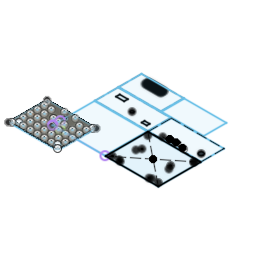
script OS 25 v11 (Autodesk Fusion 360 design; units mm, degrees)
Autodesk Fusion 360 part; units mm, degrees
(part 1 of 6)
sketch "top content" plane through (0, 0, 0) normal (0, 0, 1) x (1, 0, 0)
  circle A0 centre (59.5, 109.5) radius 1.5
  circle A1 centre (59.5, 78.5) radius 1.5
  circle A2 centre (90.5, 109.5) radius 1.5
  line L0 (0, 120) -> (150, 120) construction
  line L1 (150, 120) -> (150, 0) construction
  line L2 (150, 0) -> (0, 0) construction
  circle A3 centre (20, 20) radius 6.4
  circle A4 centre (75, 60) radius 1.588
  circle A5 centre (90.5, 78.5) radius 1.5
  circle A6 centre (75, 94) radius 11
  line L3 (0, 0) -> (0, 120) construction
  line L4 (1.75, 0) -> (22.5, 0)
  line L5 (0, 1.75) -> (0, 22.5)
  line L6 (0, 60) -> (150, 60) construction
  line L7 (75, 120) -> (75, 0) construction
  circle A7 centre (130, 20) radius 6.4
  point P0 (75, 60)
  point P1 (75, 60)
  dimension "d2090" = 31
  dimension "d2091" = 31
  dimension "d2092" = 150
  dimension "d2093" = 120
  dimension "d2094" = 12.8
  dimension "d2096" = 3
  dimension "d2104" = 15.5
  dimension "d2105" = 15.5
  dimension "d5914" = 22
  dimension "d5917" = 40
  dimension "d5918" = 55
  dimension "d5919" = 34
  constraint perpendicular L0 L1
  constraint parallel L0 L2
  constraint parallel L1 L3
  constraint coincident P1 P0
  constraint horizontal L2
  constraint collinear L2 L4
  constraint collinear L3 L5
  constraint midpoint L3 L6.start
  constraint midpoint L1 L6.end
  constraint midpoint L0 L7.start
  constraint midpoint L2 L7.end
  constraint coincident A6.centre L7
  constraint symmetric A3 L7 A7
  measures "d2092" distance of L0.start L0.end
  measures "d2093" distance of L0.start L2.end
  measures "d2094" diameter of A3
  measures "d2096" diameter of A1
  measures "d2104" horizontal distance of A6.centre A2.centre
  measures "d2105" vertical distance of A6.centre A5.centre
  measures "d5914" diameter of A6
  measures "d5917" distance of A3.centre L6
  measures "d5918" distance of A3.centre L7
  measures "d5919" distance of A6.centre L6
sketch "platform content" plane through (0, 0, 0) normal (0, 0, 1) x (1, 0, 0) in component "platform"
  circle A0 centre (55, -40) radius 6.4
  line L0 (-70, -50) -> (-70, 50)
  line L1 (-65, 55) -> (65, 55)
  line L2 (-70, 0) -> (70, 0) construction
  circle A1 centre (-15.5, 49.5) radius 1.5
  line L3 (70, 50) -> (70, -50)
  line L4 (65, -55) -> (-65, -55)
  line L5 (0, 55) -> (0, -55) construction
  circle A2 centre (-55, -40) radius 6.4
  circle A3 centre (15.5, 18.5) radius 1.5
  circle A4 centre (-15.5, 18.5) radius 1.5
  circle A5 centre (0, 34) radius 6.4
  circle A6 centre (15.5, 49.5) radius 1.5
  arc A7 (-70, -50) -> (-65, -55) centre (-65, -50) ccw
  arc A8 (65, -55) -> (70, -50) centre (65, -50) ccw
  arc A9 (70, 50) -> (65, 55) centre (65, 50) ccw
  arc A10 (-65, 55) -> (-70, 50) centre (-65, 50) ccw
  circle A11 centre (0, 0) radius 1.005
  circle A12 centre (0, -3) radius 1.5
  circle A13 centre (-40, -43) radius 1.5
  circle A14 centre (-60, -23) radius 1.5
  circle A15 centre (-60, -3) radius 1.5
  circle A16 centre (40, -43) radius 1.5
  circle A17 centre (0, -23) radius 1.5
  circle A18 centre (-20, -3) radius 1.5
  circle A19 centre (40, -3) radius 1.5
  circle A20 centre (60, -3) radius 1.5
  circle A21 centre (60, -23) radius 1.5
  circle A22 centre (-20, -43) radius 1.5
  circle A23 centre (20, -43) radius 1.5
  circle A24 centre (-40, -3) radius 1.5
  circle A25 centre (20, -3) radius 1.5
  circle A26 centre (-60, 17) radius 1.5
  circle A27 centre (-40, 17) radius 1.5
  circle A28 centre (0, 17) radius 1.5
  circle A29 centre (40, 17) radius 1.5
  circle A30 centre (60, 17) radius 1.5
  circle A31 centre (-60, 37) radius 1.5
  circle A32 centre (-40, 37) radius 1.5
  circle A33 centre (40, 37) radius 1.5
  circle A34 centre (60, 37) radius 1.5
  circle A35 centre (0, -43) radius 1.5
  circle A36 centre (-40, -23) radius 1.5
  circle A37 centre (-20, -23) radius 1.5
  circle A38 centre (20, -23) radius 1.5
  circle A39 centre (40, -23) radius 1.5
  circle A40 centre (-65, 50) radius 1.5
  circle A41 centre (65, 50) radius 1.5
  circle A42 centre (65, -50) radius 1.5
  circle A43 centre (-65, -50) radius 1.5
  point P0 (-70, -55)
  point P1 (70, 55)
  point P2 (-70, 55)
  dimension "d5927" = 31
  dimension "d5928" = 31
  dimension "d5929" = 140
  dimension "d5930" = 110
  dimension "d5931" = 12.8
  dimension "d5932" = 3
  dimension "d5933" = 15.5
  dimension "d5934" = 15.5
  dimension "d5935" = 12.8
  dimension "d5936" = 40
  dimension "d5937" = 55
  dimension "d5938" = 34
  dimension "d5939" = 5
  dimension "d5940" = 5
  dimension "d5941" = 5
  dimension "d5942" = 5
  dimension "d5943" = 2.01
  dimension "d5948" = 70
  dimension "d5959" = 3
  dimension "d5960" = 3
  dimension "d5961" = 37
  dimension "d5962" = 37
  dimension "d5965" = 20
  dimension "d5966" = 20
  dimension "d5967" = 3
  dimension "d5968" = 3
  dimension "d5969" = 3
  dimension "d5970" = 3
  constraint perpendicular L1 L3
  constraint parallel L1 L4
  constraint parallel L0 L3
  constraint horizontal L4
  constraint coincident A5.centre L5
  constraint symmetric A0 L5 A2
  constraint midpoint L5 A11.centre
  constraint coincident L2.start L0
  constraint coincident L5.end L4
  constraint coincident P0 L0
  constraint coincident P0 L4
  constraint tangent L0 A7
  constraint tangent L4 A7
  constraint coincident L2.end L3
  constraint tangent L4 A8
  constraint tangent L3 A8
  constraint coincident L5.start L1
  constraint coincident P1 L1
  constraint coincident P1 L3
  constraint tangent L1 A9
  constraint tangent L3 A9
  constraint coincident P2 L1
  constraint coincident P2 L0
  constraint tangent L1 A10
  constraint tangent L0 A10
  constraint coincident A11.centre origin
  constraint vertical L5
  constraint horizontal L2
  constraint coincident L2 A11.centre
  constraint coincident L5 A12.centre
  constraint concentric A10 A40
  constraint concentric A9 A41
  constraint concentric A8 A42
  constraint concentric A7 A43
  measures "d5929" distance of P1 P2
  measures "d5930" distance of P0 P2
  measures "d5931" diameter of A2
  measures "d5932" diameter of A4
  measures "d5933" horizontal distance of A6.centre A5.centre
  measures "d5934" vertical distance of A3.centre A5.centre
  measures "d5935" diameter of A5
  measures "d5936" distance of A2.centre L2
  measures "d5937" distance of A2.centre L5
  measures "d5938" distance of A5.centre L2
  measures "d5939" radius of A7
  measures "d5940" radius of A8
  measures "d5941" radius of A9
  measures "d5942" radius of A10
  measures "d5943" diameter of A11
  measures "d5948" distance of L3 L5
  measures "d5959" diameter of A12
  measures "d5960" distance of L2 A12.centre
  measures "d5961" vertical distance of A0.centre A12.centre
  measures "d5962" distance of A5.centre A12.centre
  measures "d5967" diameter of A40
  measures "d5968" diameter of A41
  measures "d5969" diameter of A42
  measures "d5970" diameter of A43
sketch "bottom content" plane through (0, 0, 0) normal (0, 0, 1) x (1, 0, 0)
  line L0 (302.01, 120) -> (152.01, 120)
  line L1 (152.01, 120) -> (152.01, 0)
  line L2 (152.01, 0) -> (302.01, 0)
  line L3 (302.01, 0) -> (302.01, 120)
  line L4 (302.01, 120) -> (152.01, 0) construction
  line L5 (152.01, 120) -> (302.01, 0) construction
  circle A0 centre (180.01, 10) radius 1
  circle A1 centre (161.535, 9.525) radius 1.005
  line L6 (150, 0) -> (0, 0)
  circle A2 centre (186.01, 7.175) radius 1
  circle A3 centre (268.01, 7.175) radius 1
  circle A4 centre (186.01, 69.175) radius 1
  circle A5 centre (268.01, 69.175) radius 1
  point P0 (227.01, 60)
  point P1 (274.01, 10)
  point P2 (180.01, 58)
  point P3 (274.01, 58)
  point P4 (292.485, 110.475)
  point P5 (292.485, 9.525)
  point P6 (161.535, 110.475)
  point P7 (292.485, 110.475)
  dimension "d3674" = 150
  dimension "d3675" = 120
  dimension "d3676" = 2
  dimension "d3677" = 10
  dimension "d3678" = 47
  dimension "d3681" = 94
  dimension "d3682" = 48
  dimension "d3683" = 2.01
  dimension "d3684" = 9.525
  dimension "d3685" = 9.525
  dimension "d3687" = 360
  dimension "d3690" = 130.95
  dimension "d3691" = 100.95
  dimension "d3731" = 152.01
  dimension "d5973" = 2
  dimension "d5974" = 7.175
  dimension "d5977" = 82
  dimension "d5978" = 62
  dimension "d5979" = 41
  constraint horizontal L0
  constraint perpendicular L0 L1
  constraint parallel L0 L2
  constraint parallel L1 L3
  constraint coincident L4 P0
  constraint coincident L5 P0
  constraint collinear L2 L6
  measures "d3674" distance of L1.end L2.end
  measures "d3675" distance of L0.start L2.end
  measures "d3676" diameter of A0
  measures "d3677" distance of L2 A0.centre
  measures "d3678" horizontal distance of P0 A0.centre
  measures "d3683" diameter of A1
  measures "d3684" distance of L2 A1.centre
  measures "d3685" distance of L1 A1.centre
  measures "d3731" distance of L6.end L1
  measures "d5973" diameter of A2
  measures "d5974" distance of L2 A2.centre
  measures "d5979" horizontal distance of P0 A2.centre
sketch "back content" plane through (0, 0, 0) normal (0, 0, 1) x (1, 0, 0)
  line L0 (152.01, 187.01) -> (302.01, 187.01) construction
  line L1 (302.01, 187.01) -> (302.01, 122.01) construction
  line L2 (302.01, 122.01) -> (152.01, 122.01) construction
  line L3 (152.01, 122.01) -> (152.01, 187.01) construction
  circle A0 centre (282.01, 142.01) radius 5.6
  line L4 (0, 0) -> (0, 120)
  line L5 (206.01, 128.51) -> (196.01, 128.51)
  line L6 (196.01, 128.51) -> (196.01, 138.51)
  line L7 (196.01, 138.51) -> (206.01, 138.51)
  line L8 (206.01, 138.51) -> (206.01, 128.51)
  line L9 (206.01, 128.51) -> (196.01, 138.51) construction
  line L10 (196.01, 128.51) -> (206.01, 138.51) construction
  line L11 (186.01, 128.51) -> (246, 128.51) construction
  line L12 (224.51, 139.51) -> (212.51, 139.51)
  line L13 (212.51, 139.51) -> (212.51, 128.51)
  line L14 (212.51, 128.51) -> (224.51, 128.51)
  line L15 (224.51, 128.51) -> (224.51, 139.51)
  line L16 (224.51, 139.51) -> (212.51, 128.51) construction
  line L17 (212.51, 139.51) -> (224.51, 128.51) construction
  line L18 (248.71, 128.51) -> (233.71, 128.51)
  line L19 (233.71, 128.51) -> (233.71, 131.01)
  line L20 (233.71, 131.01) -> (248.71, 131.01)
  line L21 (248.71, 131.01) -> (248.71, 128.51)
  line L22 (248.71, 128.51) -> (233.71, 131.01) construction
  line L23 (233.71, 128.51) -> (248.71, 131.01) construction
  point P0 (22.5, 0)
  point P1 (201.01, 133.51)
  point P2 (218.51, 134.01)
  point P3 (241.21, 129.76)
  dimension "d381" = 150
  dimension "d382" = 65
  dimension "d387" = 11.2
  dimension "d388" = 20
  dimension "d389" = 20
  dimension "d3694" = 152.01
  dimension "d3695" = 122.01
  dimension "d5984" = 6.5
  dimension "d5985" = 10
  dimension "d5986" = 10
  dimension "d5987" = 15
  dimension "d5988" = 12
  dimension "d5989" = 32.5
  dimension "d5990" = 11
  dimension "d5991" = 15
  dimension "d5992" = 2.5
  dimension "d5993" = 55.2
  dimension "d5995" = 34
  constraint horizontal L0
  constraint horizontal L2
  constraint vertical L3
  constraint vertical L1
  constraint horizontal L5
  constraint perpendicular L5 L6
  constraint parallel L5 L7
  constraint parallel L6 L8
  constraint coincident L9 P1
  constraint coincident L10 P1
  constraint perpendicular L6 L11
  constraint collinear L5 L11
  constraint horizontal L12
  constraint perpendicular L12 L13
  constraint parallel L12 L14
  constraint parallel L13 L15
  constraint coincident L16 P2
  constraint coincident L17 P2
  constraint collinear L11 L14
  constraint horizontal L18
  constraint perpendicular L18 L19
  constraint parallel L18 L20
  constraint parallel L19 L21
  constraint coincident L22 P3
  constraint coincident L23 P3
  constraint collinear L11 L18
  measures "d381" distance of L0.start L0.end
  measures "d382" distance of L0.start L2.end
  measures "d387" diameter of A0
  measures "d388" distance of L2 A0.centre
  measures "d389" distance of L1 A0.centre
  measures "d3694" distance of L3 L4
  measures "d3695" distance of L2 P0
  measures "d5984" distance of L2 L11
  measures "d5985" distance of L5.end L6.end
  measures "d5986" distance of L6.end L7.end
  measures "d5987" horizontal distance of P1 L11.start
  measures "d5988" distance of L13.end L14.end
  measures "d5989" horizontal distance of L11.start P2
  measures "d5990" distance of L12.start L14.end
  measures "d5991" distance of L19.end L20.end
  measures "d5992" distance of L18.start L20.end
  measures "d5993" horizontal distance of L11.start P3
  measures "d5995" horizontal distance of L2.end L11.start
sketch "front content" plane through (0, 0, 0) normal (0, 0, 1) x (1, 0, 0)
  line L0 (20, 172.01) -> (43, 172.01)
  line L1 (43, 172.01) -> (43, 161.51)
  line L2 (43, 161.51) -> (20, 161.51)
  line L3 (20, 161.51) -> (20, 172.01)
  circle A0 centre (80, 147.01) radius 3.5
  line L4 (120.5, 142.21) -> (135, 142.21)
  line L5 (135, 142.21) -> (135, 134.01)
  line L6 (135, 134.01) -> (120.5, 134.01)
  line L7 (120.5, 134.01) -> (120.5, 142.21)
  line L8 (0, 187.01) -> (150, 187.01) construction
  line L9 (150, 187.01) -> (150, 122.01) construction
  line L10 (150, 122.01) -> (0, 122.01) construction
  line L11 (0, 122.01) -> (0, 187.01) construction
  line L12 (150, 0) -> (0, 0)
  line L13 (0, 1.75) -> (0, 22.5)
  dimension "d332" = 23
  dimension "d333" = 10.5
  dimension "d336" = 7
  dimension "d339" = 14.5
  dimension "d340" = 8.2
  dimension "d371" = 150
  dimension "d372" = 65
  dimension "d374" = 20
  dimension "d376" = 15
  dimension "d377" = 12
  dimension "d378" = 15
  dimension "d379" = 25
  dimension "d380" = 70
  dimension "d3693" = 122.01
  constraint horizontal L0
  constraint vertical L1
  constraint horizontal L2
  constraint vertical L3
  constraint horizontal L4
  constraint vertical L5
  constraint horizontal L6
  constraint vertical L7
  constraint horizontal L8
  constraint vertical L9
  constraint horizontal L10
  constraint vertical L11
  constraint collinear L11 L13
  measures "d332" distance of L0.start L0.end
  measures "d333" distance of L0.start L2.end
  measures "d336" diameter of A0
  measures "d339" distance of L4.start L4.end
  measures "d340" distance of L4.start L6.end
  measures "d371" distance of L8.start L8.end
  measures "d372" distance of L8.start L10.end
  measures "d374" distance of L3 L11
  measures "d376" distance of L0 L8
  measures "d377" distance of L6 L10
  measures "d378" distance of L5 L9
  measures "d379" distance of A0.centre L10
  measures "d380" distance of A0.centre L9
  measures "d3693" distance of L10.end L12
sketch "left content" plane through (0, 0, 0) normal (0, 0, 1) x (1, 0, 0)
  line L0 (120, 254.02) -> (120, 189.02) construction
  line L1 (120, 189.02) -> (0, 189.02) construction
  line L2 (0, 189.02) -> (0, 254.02) construction
  line L3 (0, 254.02) -> (120, 254.02) construction
  line L4 (0, 1.75) -> (0, 22.5)
  circle A0 centre (30, 234.02) radius 1.005
  circle A1 centre (30, 239.02) radius 1.005
  circle A2 centre (30, 244.02) radius 1.005
  circle A3 centre (35, 234.02) radius 1.005
  circle A4 centre (40, 234.02) radius 1.005
  circle A5 centre (45, 234.02) radius 1.005
  circle A6 centre (50, 234.02) radius 1.005
  circle A7 centre (55, 234.02) radius 1.005
  circle A8 centre (60, 234.02) radius 1.005
  circle A9 centre (65, 234.02) radius 1.005
  circle A10 centre (70, 234.02) radius 1.005
  circle A11 centre (75, 234.02) radius 1.005
  circle A12 centre (35, 239.02) radius 1.005
  circle A13 centre (40, 239.02) radius 1.005
  circle A14 centre (45, 239.02) radius 1.005
  circle A15 centre (50, 239.02) radius 1.005
  circle A16 centre (55, 239.02) radius 1.005
  circle A17 centre (60, 239.02) radius 1.005
  circle A18 centre (65, 239.02) radius 1.005
  circle A19 centre (70, 239.02) radius 1.005
  circle A20 centre (75, 239.02) radius 1.005
  circle A21 centre (35, 244.02) radius 1.005
  circle A22 centre (40, 244.02) radius 1.005
  circle A23 centre (45, 244.02) radius 1.005
  circle A24 centre (50, 244.02) radius 1.005
  circle A25 centre (55, 244.02) radius 1.005
  circle A26 centre (60, 244.02) radius 1.005
  circle A27 centre (65, 244.02) radius 1.005
  circle A28 centre (70, 244.02) radius 1.005
  circle A29 centre (75, 244.02) radius 1.005
  point P0 (22.5, 0)
  dimension "d2844" = 65
  dimension "d2845" = 120
  dimension "d3696" = 189.02
  dimension "d3712" = 2.01
  dimension "d3715" = 5
  dimension "d3716" = 5
  dimension "d3717" = 30
  dimension "d3718" = 10
  constraint coincident L0.end L1.start
  constraint coincident L2.end L3.start
  constraint collinear L2 L4
  constraint horizontal L3
  constraint horizontal L1
  measures "d2844" distance of L2.end L1.end
  measures "d2845" distance of L0 L2
  measures "d3696" distance of L1 P0
  measures "d3712" diameter of A0
  measures "d3717" distance of L2 A0.centre
  measures "d3718" distance of L3 A2.centre
sketch "right content" plane through (0, 0, 0) normal (0, 0, 1) x (1, 0, 0)
  circle A0 centre (157.01, 239.02) radius 1.005
  line L0 (122.01, 189.02) -> (122.01, 254.02) construction
  circle A1 centre (162.01, 244.02) radius 1.005
  circle A2 centre (172.01, 244.02) radius 1.005
  circle A3 centre (162.01, 234.02) radius 1.005
  circle A4 centre (192.01, 239.02) radius 1.005
  circle A5 centre (157.01, 234.02) radius 1.005
  circle A6 centre (152.01, 244.02) radius 1.005
  line L1 (122.01, 254.02) -> (242.01, 254.02) construction
  circle A7 centre (197.01, 239.02) radius 1.005
  circle A8 centre (167.01, 234.02) radius 1.005
  circle A9 centre (187.01, 244.02) radius 1.005
  circle A10 centre (152.01, 234.02) radius 1.005
  circle A11 centre (162.01, 239.02) radius 1.005
  line L2 (242.01, 254.02) -> (242.01, 189.02) construction
  circle A12 centre (197.01, 244.02) radius 1.005
  line L3 (242.01, 189.02) -> (122.01, 189.02) construction
  circle A13 centre (197.01, 234.02) radius 1.005
  circle A14 centre (182.01, 239.02) radius 1.005
  circle A15 centre (187.01, 239.02) radius 1.005
  circle A16 centre (172.01, 239.02) radius 1.005
  circle A17 centre (182.01, 244.02) radius 1.005
  circle A18 centre (177.01, 239.02) radius 1.005
  circle A19 centre (152.01, 239.02) radius 1.005
  circle A20 centre (177.01, 244.02) radius 1.005
  circle A21 centre (167.01, 244.02) radius 1.005
  circle A22 centre (157.01, 244.02) radius 1.005
  circle A23 centre (192.01, 244.02) radius 1.005
  circle A24 centre (187.01, 234.02) radius 1.005
  circle A25 centre (192.01, 234.02) radius 1.005
  circle A26 centre (177.01, 234.02) radius 1.005
  circle A27 centre (182.01, 234.02) radius 1.005
  circle A28 centre (167.01, 239.02) radius 1.005
  circle A29 centre (172.01, 234.02) radius 1.005
  dimension "d3723" = 5
  dimension "d3724" = 5
  dimension "d3726" = 120
  dimension "d3727" = 2.01
  dimension "d3728" = 30
  dimension "d3729" = 10
  dimension "d3730" = 65
  dimension "d5980" = 189.02
  dimension "d5981" = 122.01
  constraint coincident L2.end L3.start
  constraint coincident L0.end L1.start
  constraint horizontal L1
  constraint horizontal L3
  constraint vertical L2
  measures "d3726" distance of L0 L2
  measures "d3727" diameter of A10
  measures "d3728" distance of A10.centre L0
  measures "d3729" distance of A6.centre L1
  measures "d3730" distance of L1 L3
  measures "d5980" vertical distance of origin L0.start
  measures "d5981" horizontal distance of origin L0.end
sketch "b  stock" plane through (0, 0, 0) normal (0, 0, 1) x (1, 0, 0)
  line L0 (0, 0) -> (304.8, 0)
  line L1 (304.8, 0) -> (304.8, 609.6)
  line L2 (304.8, 609.6) -> (0, 609.6)
  line L3 (0, 609.6) -> (0, 0)
extrude "b  stock body extrude" add sketch "b  stock" along normal blind 3.175 makes body 1
sketch "b  layout" plane through (0, 0, 0) normal (0, 0, 1) x (1, 0, 0)
  line L0 (0, 0) -> (150, 0)
  line L1 (150, 0) -> (150, 120)
  line L2 (150, 120) -> (0, 120)
  line L3 (0, 120) -> (0, 0)
  line L4 (152.01, 0) -> (302.01, 0)
  line L5 (302.01, 0) -> (302.01, 120)
  line L6 (302.01, 120) -> (152.01, 120)
  line L7 (152.01, 120) -> (152.01, 0)
  line L8 (0, 122.01) -> (150, 122.01)
  line L9 (150, 122.01) -> (150, 187.01)
  line L10 (150, 187.01) -> (0, 187.01)
  line L11 (0, 187.01) -> (0, 122.01)
  line L12 (152.01, 122.01) -> (302.01, 122.01)
  line L13 (302.01, 122.01) -> (302.01, 187.01)
  line L14 (302.01, 187.01) -> (152.01, 187.01)
  line L15 (152.01, 187.01) -> (152.01, 122.01)
  line L16 (0, 189.02) -> (120, 189.02)
  line L17 (120, 189.02) -> (120, 254.02)
  line L18 (120, 254.02) -> (0, 254.02)
  line L19 (0, 254.02) -> (0, 189.02)
  line L20 (122.01, 189.02) -> (242.01, 189.02)
  line L21 (242.01, 189.02) -> (242.01, 254.02)
  line L22 (242.01, 254.02) -> (122.01, 254.02)
  line L23 (122.01, 254.02) -> (122.01, 189.02)
sketch "b top lines" plane through (0, 0, 0) normal (0, 0, 1) x (1, 0, 0) in component "b top component"
  line L0 (0, 0) -> (10.08, 0)
  line L1 (10.08, 0) -> (10.08, 3.175)
  line L2 (10.08, 3.175) -> (19.92, 3.175)
  line L3 (19.92, 3.175) -> (19.92, 0)
  line L4 (19.92, 0) -> (30.08, 0)
  line L5 (30.08, 0) -> (30.08, 3.175)
  line L6 (30.08, 3.175) -> (39.92, 3.175)
  line L7 (39.92, 3.175) -> (39.92, 0)
  line L8 (39.92, 0) -> (50.08, 0)
  line L9 (50.08, 0) -> (50.08, 3.175)
  line L10 (50.08, 3.175) -> (59.92, 3.175)
  line L11 (59.92, 3.175) -> (59.92, 0)
  line L12 (59.92, 0) -> (70.08, 0)
  line L13 (70.08, 0) -> (70.08, 3.175)
  line L14 (70.08, 3.175) -> (79.92, 3.175)
  line L15 (79.92, 3.175) -> (79.92, 0)
  line L16 (79.92, 0) -> (90.08, 0)
  line L17 (90.08, 0) -> (90.08, 3.175)
  line L18 (90.08, 3.175) -> (99.92, 3.175)
  line L19 (99.92, 3.175) -> (99.92, 0)
  line L20 (99.92, 0) -> (110.08, 0)
  line L21 (110.08, 0) -> (110.08, 3.175)
  line L22 (110.08, 3.175) -> (119.92, 3.175)
  line L23 (119.92, 3.175) -> (119.92, 0)
  line L24 (119.92, 0) -> (130.08, 0)
  line L25 (130.08, 0) -> (130.08, 3.175)
  line L26 (130.08, 3.175) -> (139.92, 3.175)
  line L27 (139.92, 3.175) -> (139.92, 0)
  line L28 (139.92, 0) -> (150, 0)
  line L29 (150, 0) -> (150, 15.08)
  line L30 (150, 15.08) -> (146.825, 15.08)
  line L31 (146.825, 15.08) -> (146.825, 24.92)
  line L32 (146.825, 24.92) -> (150, 24.92)
  line L33 (150, 24.92) -> (150, 35.08)
  line L34 (150, 35.08) -> (146.825, 35.08)
  line L35 (146.825, 35.08) -> (146.825, 44.92)
  line L36 (146.825, 44.92) -> (150, 44.92)
  line L37 (150, 44.92) -> (150, 55.08)
  line L38 (150, 55.08) -> (146.825, 55.08)
  line L39 (146.825, 55.08) -> (146.825, 64.92)
  line L40 (146.825, 64.92) -> (150, 64.92)
  line L41 (150, 64.92) -> (150, 75.08)
  line L42 (150, 75.08) -> (146.825, 75.08)
  line L43 (146.825, 75.08) -> (146.825, 84.92)
  line L44 (146.825, 84.92) -> (150, 84.92)
  line L45 (150, 84.92) -> (150, 95.08)
  line L46 (150, 95.08) -> (146.825, 95.08)
  line L47 (146.825, 95.08) -> (146.825, 104.92)
  line L48 (146.825, 104.92) -> (150, 104.92)
  line L49 (150, 104.92) -> (150, 120)
  line L50 (0, 120) -> (10.08, 120)
  line L51 (10.08, 120) -> (10.08, 116.825)
  line L52 (10.08, 116.825) -> (19.92, 116.825)
  line L53 (19.92, 116.825) -> (19.92, 120)
  line L54 (19.92, 120) -> (30.08, 120)
  line L55 (30.08, 120) -> (30.08, 116.825)
  line L56 (30.08, 116.825) -> (39.92, 116.825)
  line L57 (39.92, 116.825) -> (39.92, 120)
  line L58 (39.92, 120) -> (50.08, 120)
  line L59 (50.08, 120) -> (50.08, 116.825)
  line L60 (50.08, 116.825) -> (59.92, 116.825)
  line L61 (59.92, 116.825) -> (59.92, 120)
  line L62 (59.92, 120) -> (70.08, 120)
  line L63 (70.08, 120) -> (70.08, 116.825)
  line L64 (70.08, 116.825) -> (79.92, 116.825)
  line L65 (79.92, 116.825) -> (79.92, 120)
  line L66 (79.92, 120) -> (90.08, 120)
  line L67 (90.08, 120) -> (90.08, 116.825)
  line L68 (90.08, 116.825) -> (99.92, 116.825)
  line L69 (99.92, 116.825) -> (99.92, 120)
  line L70 (99.92, 120) -> (110.08, 120)
  line L71 (110.08, 120) -> (110.08, 116.825)
  line L72 (110.08, 116.825) -> (119.92, 116.825)
  line L73 (119.92, 116.825) -> (119.92, 120)
  line L74 (119.92, 120) -> (130.08, 120)
  line L75 (130.08, 120) -> (130.08, 116.825)
  line L76 (130.08, 116.825) -> (139.92, 116.825)
  line L77 (139.92, 116.825) -> (139.92, 120)
  line L78 (139.92, 120) -> (150, 120)
  line L79 (0, 0) -> (0, 15.08)
  line L80 (0, 15.08) -> (3.175, 15.08)
  line L81 (3.175, 15.08) -> (3.175, 24.92)
  line L82 (3.175, 24.92) -> (0, 24.92)
  line L83 (0, 24.92) -> (0, 35.08)
  line L84 (0, 35.08) -> (3.175, 35.08)
  line L85 (3.175, 35.08) -> (3.175, 44.92)
  line L86 (3.175, 44.92) -> (0, 44.92)
  line L87 (0, 44.92) -> (0, 55.08)
  line L88 (0, 55.08) -> (3.175, 55.08)
  line L89 (3.175, 55.08) -> (3.175, 64.92)
  line L90 (3.175, 64.92) -> (0, 64.92)
  line L91 (0, 64.92) -> (0, 75.08)
  line L92 (0, 75.08) -> (3.175, 75.08)
  line L93 (3.175, 75.08) -> (3.175, 84.92)
  line L94 (3.175, 84.92) -> (0, 84.92)
  line L95 (0, 84.92) -> (0, 95.08)
  line L96 (0, 95.08) -> (3.175, 95.08)
  line L97 (3.175, 95.08) -> (3.175, 104.92)
  line L98 (3.175, 104.92) -> (0, 104.92)
  line L99 (0, 104.92) -> (0, 120)
  dimension "d5190" = 10.08
  dimension "d5191" = 3.175
  dimension "d5192" = 9.84
  dimension "d5193" = 3.175
  dimension "d5194" = 10.16
  dimension "d5195" = 3.175
  dimension "d5196" = 9.84
  dimension "d5197" = 3.175
  dimension "d5198" = 10.16
  dimension "d5199" = 3.175
  dimension "d5200" = 9.84
  dimension "d5201" = 3.175
  dimension "d5202" = 10.16
  dimension "d5203" = 3.175
  dimension "d5204" = 9.84
  dimension "d5205" = 3.175
  dimension "d5206" = 10.16
  dimension "d5207" = 3.175
  dimension "d5208" = 9.84
  dimension "d5209" = 3.175
  dimension "d5210" = 10.16
  dimension "d5211" = 3.175
  dimension "d5212" = 9.84
  dimension "d5213" = 3.175
  dimension "d5214" = 10.16
  dimension "d5215" = 3.175
  dimension "d5216" = 9.84
  dimension "d5217" = 3.175
  dimension "d5218" = 10.08
  dimension "d5233" = 15.08
  dimension "d5234" = 3.175
  dimension "d5235" = 9.84
  dimension "d5236" = 3.175
  dimension "d5237" = 10.16
  dimension "d5238" = 3.175
  dimension "d5239" = 9.84
  dimension "d5240" = 3.175
  dimension "d5241" = 10.16
  dimension "d5242" = 3.175
  dimension "d5243" = 9.84
  dimension "d5244" = 3.175
  dimension "d5245" = 10.16
  dimension "d5246" = 3.175
  dimension "d5247" = 9.84
  dimension "d5248" = 3.175
  dimension "d5249" = 10.16
  dimension "d5250" = 3.175
  dimension "d5251" = 9.84
  dimension "d5252" = 3.175
  dimension "d5253" = 15.08
  dimension "d5264" = 10.08
  dimension "d5265" = 3.175
  dimension "d5266" = 9.84
  dimension "d5267" = 3.175
  dimension "d5268" = 10.16
  dimension "d5269" = 3.175
  dimension "d5270" = 9.84
  dimension "d5271" = 3.175
  dimension "d5272" = 10.16
  dimension "d5273" = 3.175
  dimension "d5274" = 9.84
  dimension "d5275" = 3.175
  dimension "d5276" = 10.16
  dimension "d5277" = 3.175
  dimension "d5278" = 9.84
  dimension "d5279" = 3.175
  dimension "d5280" = 10.16
  dimension "d5281" = 3.175
  dimension "d5282" = 9.84
  dimension "d5283" = 3.175
  dimension "d5284" = 10.16
  dimension "d5285" = 3.175
  dimension "d5286" = 9.84
  dimension "d5287" = 3.175
  dimension "d5288" = 10.16
  dimension "d5289" = 3.175
  dimension "d5290" = 9.84
  dimension "d5291" = 3.175
  dimension "d5292" = 10.08
  dimension "d5307" = 15.08
  dimension "d5308" = 3.175
  dimension "d5309" = 9.84
  dimension "d5310" = 3.175
  dimension "d5311" = 10.16
  dimension "d5312" = 3.175
  dimension "d5313" = 9.84
  dimension "d5314" = 3.175
  dimension "d5315" = 10.16
  dimension "d5316" = 3.175
  dimension "d5317" = 9.84
  dimension "d5318" = 3.175
  dimension "d5319" = 10.16
  dimension "d5320" = 3.175
  dimension "d5321" = 9.84
  dimension "d5322" = 3.175
  dimension "d5323" = 10.16
  dimension "d5324" = 3.175
  dimension "d5325" = 9.84
  dimension "d5326" = 3.175
  dimension "d5327" = 15.08
  constraint horizontal L0
  constraint vertical L1
  constraint horizontal L2
  constraint vertical L3
  constraint horizontal L4
  constraint vertical L5
  constraint horizontal L6
  constraint vertical L7
  constraint horizontal L8
  constraint vertical L9
  constraint horizontal L10
  constraint vertical L11
  constraint horizontal L12
  constraint vertical L13
  constraint horizontal L14
  constraint vertical L15
  constraint horizontal L16
  constraint vertical L17
  constraint horizontal L18
  constraint vertical L19
  constraint horizontal L20
  constraint vertical L21
  constraint horizontal L22
  constraint vertical L23
  constraint horizontal L24
  constraint vertical L25
  constraint horizontal L26
  constraint vertical L27
  constraint horizontal L28
  constraint vertical L29
  constraint horizontal L30
  constraint vertical L31
  constraint horizontal L32
  constraint vertical L33
  constraint horizontal L34
  constraint vertical L35
  constraint horizontal L36
  constraint vertical L37
  constraint horizontal L38
  constraint vertical L39
  constraint horizontal L40
  constraint vertical L41
  constraint horizontal L42
  constraint vertical L43
  constraint horizontal L44
  constraint vertical L45
  constraint horizontal L46
  constraint vertical L47
  constraint horizontal L48
  constraint vertical L49
  constraint horizontal L50
  constraint vertical L51
  constraint horizontal L52
  constraint vertical L53
  constraint horizontal L54
  constraint vertical L55
  constraint horizontal L56
  constraint vertical L57
  constraint horizontal L58
  constraint vertical L59
  constraint horizontal L60
  constraint vertical L61
  constraint horizontal L62
  constraint vertical L63
  constraint horizontal L64
  constraint vertical L65
  constraint horizontal L66
  constraint vertical L67
  constraint horizontal L68
  constraint vertical L69
  constraint horizontal L70
  constraint vertical L71
  constraint horizontal L72
  constraint vertical L73
  constraint horizontal L74
  constraint vertical L75
  constraint horizontal L76
  constraint vertical L77
  constraint horizontal L78
  constraint vertical L79
  constraint horizontal L80
  constraint vertical L81
  constraint horizontal L82
  constraint vertical L83
  constraint horizontal L84
  constraint vertical L85
  constraint horizontal L86
  constraint vertical L87
  constraint horizontal L88
  constraint vertical L89
  constraint horizontal L90
  constraint vertical L91
  constraint horizontal L92
  constraint vertical L93
  constraint horizontal L94
  constraint vertical L95
  constraint horizontal L96
  constraint vertical L97
  constraint horizontal L98
  constraint vertical L99
  measures "d5190" distance of L0.start L0.end
  measures "d5191" distance of L0.end L1.end
  measures "d5192" distance of L1.end L2.end
  measures "d5193" distance of L2.end L3.end
  measures "d5194" distance of L3.end L4.end
  measures "d5195" distance of L4.end L5.end
  measures "d5196" distance of L5.end L6.end
  measures "d5197" distance of L6.end L7.end
  measures "d5198" distance of L7.end L8.end
  measures "d5199" distance of L8.end L9.end
  measures "d5200" distance of L9.end L10.end
  measures "d5201" distance of L10.end L11.end
  measures "d5202" distance of L11.end L12.end
  measures "d5203" distance of L12.end L13.end
  measures "d5204" distance of L13.end L14.end
  measures "d5205" distance of L14.end L15.end
  measures "d5206" distance of L15.end L16.end
  measures "d5207" distance of L16.end L17.end
  measures "d5208" distance of L17.end L18.end
  measures "d5209" distance of L18.end L19.end
  measures "d5210" distance of L19.end L20.end
  measures "d5211" distance of L20.end L21.end
  measures "d5212" distance of L21.end L22.end
  measures "d5213" distance of L22.end L23.end
  measures "d5214" distance of L23.end L24.end
  measures "d5215" distance of L24.end L25.end
  measures "d5216" distance of L25.end L26.end
  measures "d5217" distance of L26.end L27.end
  measures "d5218" distance of L27.end L28.end
  measures "d5233" distance of L28.end L29.end
  measures "d5234" distance of L29.end L30.end
  measures "d5235" distance of L30.end L31.end
  measures "d5236" distance of L31.end L32.end
  measures "d5237" distance of L32.end L33.end
  measures "d5238" distance of L33.end L34.end
  measures "d5239" distance of L34.end L35.end
  measures "d5240" distance of L35.end L36.end
  measures "d5241" distance of L36.end L37.end
  measures "d5242" distance of L37.end L38.end
  measures "d5243" distance of L38.end L39.end
  measures "d5244" distance of L39.end L40.end
  measures "d5245" distance of L40.end L41.end
  measures "d5246" distance of L41.end L42.end
  measures "d5247" distance of L42.end L43.end
  measures "d5248" distance of L43.end L44.end
  measures "d5249" distance of L44.end L45.end
  measures "d5250" distance of L45.end L46.end
  measures "d5251" distance of L46.end L47.end
  measures "d5252" distance of L47.end L48.end
  measures "d5253" distance of L48.end L49.end
  measures "d5264" distance of L50.start L50.end
  measures "d5265" distance of L50.end L51.end
  measures "d5266" distance of L51.end L52.end
  measures "d5267" distance of L52.end L53.end
  measures "d5268" distance of L53.end L54.end
  measures "d5269" distance of L54.end L55.end
  measures "d5270" distance of L55.end L56.end
  measures "d5271" distance of L56.end L57.end
  measures "d5272" distance of L57.end L58.end
  measures "d5273" distance of L58.end L59.end
  measures "d5274" distance of L59.end L60.end
  measures "d5275" distance of L60.end L61.end
  measures "d5276" distance of L61.end L62.end
  measures "d5277" distance of L62.end L63.end
  measures "d5278" distance of L63.end L64.end
  measures "d5279" distance of L64.end L65.end
  measures "d5280" distance of L65.end L66.end
  measures "d5281" distance of L66.end L67.end
  measures "d5282" distance of L67.end L68.end
  measures "d5283" distance of L68.end L69.end
  measures "d5284" distance of L69.end L70.end
  measures "d5285" distance of L70.end L71.end
  measures "d5286" distance of L71.end L72.end
  measures "d5287" distance of L72.end L73.end
  measures "d5288" distance of L73.end L74.end
  measures "d5289" distance of L74.end L75.end
  measures "d5290" distance of L75.end L76.end
  measures "d5291" distance of L76.end L77.end
  measures "d5292" distance of L49.end L77.end
  measures "d5307" distance of L0.start L79.end
  measures "d5308" distance of L79.end L80.end
  measures "d5309" distance of L80.end L81.end
  measures "d5310" distance of L81.end L82.end
  measures "d5311" distance of L82.end L83.end
  measures "d5312" distance of L83.end L84.end
  measures "d5313" distance of L84.end L85.end
  measures "d5314" distance of L85.end L86.end
  measures "d5315" distance of L86.end L87.end
  measures "d5316" distance of L87.end L88.end
  measures "d5317" distance of L88.end L89.end
  measures "d5318" distance of L89.end L90.end
  measures "d5319" distance of L90.end L91.end
  measures "d5320" distance of L91.end L92.end
  measures "d5321" distance of L92.end L93.end
  measures "d5322" distance of L93.end L94.end
  measures "d5323" distance of L94.end L95.end
  measures "d5324" distance of L95.end L96.end
  measures "d5325" distance of L96.end L97.end
  measures "d5326" distance of L97.end L98.end
  measures "d5327" distance of L50.start L98.end
sketch "b top circles" plane through (0, 0, 0) normal (0, 0, 1) x (1, 0, 0) in component "b top component"
  line L0 (0, 0) -> (150, 0)
  line L1 (150, 0) -> (150, 120)
  line L2 (150, 120) -> (0, 120)
  line L3 (0, 120) -> (0, 0)
  circle A0 centre (10.6946, 2.3644) radius 1.005
  circle A1 centre (19.3054, 2.3644) radius 1.005
  circle A2 centre (30.6946, 2.3644) radius 1.005
  circle A3 centre (39.3054, 2.3644) radius 1.005
  circle A4 centre (50.6946, 2.3644) radius 1.005
  circle A5 centre (59.3054, 2.3644) radius 1.005
  circle A6 centre (70.6946, 2.3644) radius 1.005
  circle A7 centre (79.3054, 2.3644) radius 1.005
  circle A8 centre (90.6946, 2.3644) radius 1.005
  circle A9 centre (99.3054, 2.3644) radius 1.005
  circle A10 centre (110.6946, 2.3644) radius 1.005
  circle A11 centre (119.3054, 2.3644) radius 1.005
  circle A12 centre (130.6946, 2.3644) radius 1.005
  circle A13 centre (139.3054, 2.3644) radius 1.005
  circle A14 centre (147.6356, 15.6946) radius 1.005
  circle A15 centre (147.6356, 24.3054) radius 1.005
  circle A16 centre (147.6356, 35.6946) radius 1.005
  circle A17 centre (147.6356, 44.3054) radius 1.005
  circle A18 centre (147.6356, 55.6946) radius 1.005
  circle A19 centre (147.6356, 64.3054) radius 1.005
  circle A20 centre (147.6356, 75.6946) radius 1.005
  circle A21 centre (147.6356, 84.3054) radius 1.005
  circle A22 centre (147.6356, 95.6946) radius 1.005
  circle A23 centre (147.6356, 104.3054) radius 1.005
  circle A24 centre (10.6946, 117.6356) radius 1.005
  circle A25 centre (19.3054, 117.6356) radius 1.005
  circle A26 centre (30.6946, 117.6356) radius 1.005
  circle A27 centre (39.3054, 117.6356) radius 1.005
  circle A28 centre (50.6946, 117.6356) radius 1.005
  circle A29 centre (59.3054, 117.6356) radius 1.005
  circle A30 centre (70.6946, 117.6356) radius 1.005
  circle A31 centre (79.3054, 117.6356) radius 1.005
  circle A32 centre (90.6946, 117.6356) radius 1.005
  circle A33 centre (99.3054, 117.6356) radius 1.005
  circle A34 centre (110.6946, 117.6356) radius 1.005
  circle A35 centre (119.3054, 117.6356) radius 1.005
  circle A36 centre (130.6946, 117.6356) radius 1.005
  circle A37 centre (139.3054, 117.6356) radius 1.005
  circle A38 centre (2.3644, 15.6946) radius 1.005
  circle A39 centre (2.3644, 24.3054) radius 1.005
  circle A40 centre (2.3644, 35.6946) radius 1.005
  circle A41 centre (2.3644, 44.3054) radius 1.005
  circle A42 centre (2.3644, 55.6946) radius 1.005
  circle A43 centre (2.3644, 64.3054) radius 1.005
  circle A44 centre (2.3644, 75.6946) radius 1.005
  circle A45 centre (2.3644, 84.3054) radius 1.005
  circle A46 centre (2.3644, 95.6946) radius 1.005
  circle A47 centre (2.3644, 104.3054) radius 1.005
  dimension "d5219" = 2.01
  dimension "d5220" = 2.01
  dimension "d5221" = 2.01
  dimension "d5222" = 2.01
  dimension "d5223" = 2.01
  dimension "d5224" = 2.01
  dimension "d5225" = 2.01
  dimension "d5226" = 2.01
  dimension "d5227" = 2.01
  dimension "d5228" = 2.01
  dimension "d5229" = 2.01
  dimension "d5230" = 2.01
  dimension "d5231" = 2.01
  dimension "d5232" = 2.01
  dimension "d5254" = 2.01
  dimension "d5255" = 2.01
  dimension "d5256" = 2.01
  dimension "d5257" = 2.01
  dimension "d5258" = 2.01
  dimension "d5259" = 2.01
  dimension "d5260" = 2.01
  dimension "d5261" = 2.01
  dimension "d5262" = 2.01
  dimension "d5263" = 2.01
  dimension "d5293" = 2.01
  dimension "d5294" = 2.01
  dimension "d5295" = 2.01
  dimension "d5296" = 2.01
  dimension "d5297" = 2.01
  dimension "d5298" = 2.01
  dimension "d5299" = 2.01
  dimension "d5300" = 2.01
  dimension "d5301" = 2.01
  dimension "d5302" = 2.01
  dimension "d5303" = 2.01
  dimension "d5304" = 2.01
  dimension "d5305" = 2.01
  dimension "d5306" = 2.01
  dimension "d5328" = 2.01
  dimension "d5329" = 2.01
  dimension "d5330" = 2.01
  dimension "d5331" = 2.01
  dimension "d5332" = 2.01
  dimension "d5333" = 2.01
  dimension "d5334" = 2.01
  dimension "d5335" = 2.01
  dimension "d5336" = 2.01
  dimension "d5337" = 2.01
  measures "d5219" diameter of A0
  measures "d5220" diameter of A1
  measures "d5221" diameter of A2
  measures "d5222" diameter of A3
  measures "d5223" diameter of A4
  measures "d5224" diameter of A5
  measures "d5225" diameter of A6
  measures "d5226" diameter of A7
  measures "d5227" diameter of A8
  measures "d5228" diameter of A9
  measures "d5229" diameter of A10
  measures "d5230" diameter of A11
  measures "d5231" diameter of A12
  measures "d5232" diameter of A13
  measures "d5254" diameter of A14
  measures "d5255" diameter of A15
  measures "d5256" diameter of A16
  measures "d5257" diameter of A17
  measures "d5258" diameter of A18
  measures "d5259" diameter of A19
  measures "d5260" diameter of A20
  measures "d5261" diameter of A21
  measures "d5262" diameter of A22
  measures "d5263" diameter of A23
  measures "d5293" diameter of A24
  measures "d5294" diameter of A25
  measures "d5295" diameter of A26
  measures "d5296" diameter of A27
  measures "d5297" diameter of A28
  measures "d5298" diameter of A29
  measures "d5299" diameter of A30
  measures "d5300" diameter of A31
  measures "d5301" diameter of A32
  measures "d5302" diameter of A33
  measures "d5303" diameter of A34
  measures "d5304" diameter of A35
  measures "d5305" diameter of A36
  measures "d5306" diameter of A37
  measures "d5328" diameter of A38
  measures "d5329" diameter of A39
  measures "d5330" diameter of A40
  measures "d5331" diameter of A41
  measures "d5332" diameter of A42
  measures "d5333" diameter of A43
  measures "d5334" diameter of A44
  measures "d5335" diameter of A45
  measures "d5336" diameter of A46
  measures "d5337" diameter of A47
extrude "b top lines body extrude" add sketch "b top lines" along normal blind 3.175 separate body makes body 2 in component "b top component"
extrude "b top circles extrude" add sketch "b top circles" along normal blind 3.175 separate body makes body 3 in component "b top component"
combine "b top lines final combine feature" operation intersect target body 2 tool bodies 3 in component "b top component"